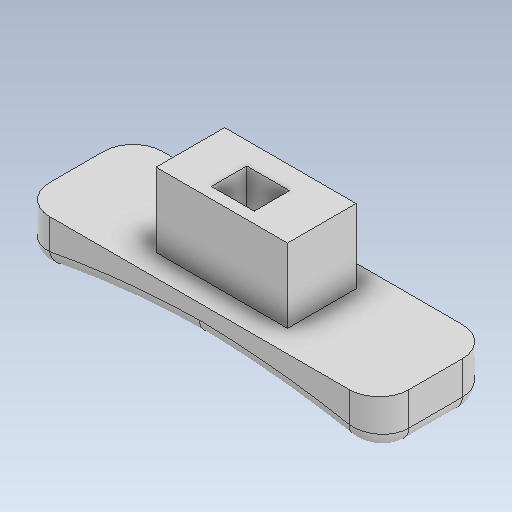
# Autodesk Inventor part: Power Switch Cap
Saved by Autodesk Inventor 2020 (Build 240168000, 168)
## iProperties
Created: 2021-06-12
Part Number: Power Switch Cap
Material: Generic
Document SubType Name: Modeling
Designer: Luke
Density: 1 g/cm^3
Appearance: Default
Author: Luke
Autodesk Inventor part; units mm, degrees
ref_plane "YZ Plane" through (0, 0, 0) normal (1, 0, 0) x (0, 1, 0)
sketch "Sketch3" plane through (0, 0, 0) normal (0, 1, 0) x (-1, 0, 0)
  line L0 (-64.0219, -58.8656) -> (-65.2719, -58.8656) projected
  line L1 (-65.2719, -58.8656) -> (-65.2719, -59.8656) projected
  line L2 (-65.2719, -59.8656) -> (-64.0219, -59.8656) projected
  line L3 (-64.0219, -59.8656) -> (-64.0219, -58.8656) projected
  line L4 (-63.9219, -59.9656) -> (-65.3719, -59.9656)
  line L5 (-65.3719, -59.9656) -> (-65.3719, -58.7656)
  line L6 (-65.3719, -58.7656) -> (-63.9219, -58.7656)
  line L7 (-63.9219, -58.7656) -> (-63.9219, -59.9656)
  line L8 (-66.8719, -60.7156) -> (-62.4219, -60.7156)
  line L9 (-62.4219, -60.7156) -> (-62.4219, -58.3956)
  line L10 (-62.4219, -58.3956) -> (-66.8719, -58.3956)
  line L11 (-66.8719, -58.3956) -> (-66.8719, -60.7156)
  line L12 (-70.1719, -61.0956) -> (-70.1719, -58.0956) projected
  line L13 (-70.1719, -58.0956) -> (-60.6119, -58.0956) projected
  line L14 (-60.6119, -61.0956) -> (-60.6119, -58.0956) projected
  dimension "d4" = 0.1
  dimension "d8" = 1.5
  dimension "d9" = 1.5
  dimension "d10" = 0.3
  dimension "d11" = 0.75
  constraints: 16 end point, 3 other
  measures "d4" distance between parallel lines of L2 L4
  measures "d8" distance between parallel lines of L9 L7
  measures "d9" distance between parallel lines of L11 L5
  measures "d10" distance between parallel lines of L13 L10
  measures "d11" distance between parallel lines of L4 L8
extrude "Extrusion3" add sketch "Sketch3" along normal blind 2.5 contours L11 L10 L9 L8
ref_plane "Work Plane1" through (65.3719, 0, -59.3656) normal (0, 0, -1) x (-1, 0, 0)
ref_plane "Work Plane2" through (64.6469, 0, -58.7656) normal (1, 0, 0) x (0, 0, -1)
sketch "Sketch4" plane through (0, 0, 0) normal (0, -1, 0) x (1, 0, 0)
  line L0 (60.1219, -61.0956) -> (60.1219, -58.0956) projected
  line L1 (67.6819, -58.0956) -> (67.6819, -61.0956) projected
  line L2 (60.1219, -58.0956) -> (67.6819, -58.0956) projected
  line L3 (62.4219, -58.3956) -> (66.8719, -58.3956) projected
  line L4 (66.8719, -58.3956) -> (66.8719, -60.7156) projected
  line L5 (66.8719, -60.7156) -> (62.4219, -60.7156) projected
  line L6 (62.4219, -60.7156) -> (62.4219, -58.3956) projected
  line L7 (70.7219, -57.6456) -> (58.5719, -57.6456)
  line L8 (58.5719, -57.6456) -> (58.5719, -61.4656)
  line L9 (58.5719, -61.4656) -> (70.7219, -61.4656)
  line L10 (70.7219, -61.4656) -> (70.7219, -57.6456)
  dimension "d13" = 3.85
  dimension "d14" = 3.85
  constraints: 8 end point
  measures "d13" distance between parallel lines of L8 L6
  measures "d14" distance between parallel lines of L10 L4
extrude "Extrusion4" add sketch "Sketch4" along normal blind 1 contours L3 L4 L5 L6 | L10 L9 L8 L7
fillet "Fillet1" radius 1 4 edges at (70.7219, -0.5, -61.4656) (58.5719, -0.5, -61.4656) (58.5719, -0.5, -57.6456) (70.7219, -0.5, -57.6456)
sketch "Sketch6" plane through (69.7219, 0, -61.4656) normal (0, 0, -1) x (-1, 0, 0)
  line L0 (10.15, -1) -> (0, -1) projected
  line L1 (11.15, -1) -> (10.15, -1) projected
  line L2 (0, -1) -> (-1, -1) projected
  line L3 (11.15, -1) -> (11.15, -1.75)
  line L4 (0, -1) -> (10.15, -1) projected
  line L5 (5.075, -1) -> (5.075, -2.2009)
  arc A0 (11.15, -1.75) -> (5.075, -1) centre (4.574, -30.0368) ccw
  line L6 (-1, -1) -> (-1, -1.75)
  arc A1 (5.075, -1) -> (-1, -1.75) centre (5.576, -30.0368) ccw
  dimension "d18" = 0.75
  constraints: 6 end point, 4 point on circle, 2 centre point, 2 symmetric about line, 2 vertical, 1 midpoint, 1 other
  measures "d18" distance of L1.start L3.end
extrude "Extrusion5" add sketch "Sketch6" against normal up to surface (3.82 mm away)
sketch "Sketch7" plane through (69.7219, -1, -61.4656) normal (0, 1, 0) x (1, 0, 0)
  arc A0 (0, -3.82) -> (1, -2.82) centre (0, -2.82) ccw projected
  line L0 (0, -3.82) -> (1, -3.82) projected
  line L1 (1, -2.82) -> (1, -3.82) projected
  arc A1 (1, -1) -> (0, 0) centre (0, -1) ccw projected
  line L2 (1, 0) -> (1, -1) projected
  line L3 (0, 0) -> (1, 0) projected
  arc A2 (-10.15, 0) -> (-11.15, -1) centre (-10.15, -1) ccw projected
  line L4 (-11.15, 0) -> (-10.15, 0) projected
  line L5 (-11.15, 0) -> (-11.15, -1) projected
  arc A3 (-11.15, -2.82) -> (-10.15, -3.82) centre (-10.15, -2.82) ccw projected
  line L6 (-11.15, -2.82) -> (-11.15, -3.82) projected
  line L7 (-11.15, -3.82) -> (-10.15, -3.82) projected
extrude "Extrusion6" cut sketch "Sketch7" against normal blind 1
fillet "Fillet2" radius 0.5 6 edges at (58.5719, -1.75, -59.5556) (62.0976, -1.1563, -57.6456) (62.0976, -1.1563, -61.4656) (70.7219, -1.75, -59.5556) (67.1962, -1.1563, -57.6456) (67.1962, -1.1563, -61.4656)
body "Solid2"
